test Acryl circle 2 mm cutter_v5 (Autodesk Fusion 360 design; units mm, degrees)
Autodesk Fusion 360 part; units mm, degrees
sketch "movingPlatform" plane through (0, 0, 0) normal (0, 0, 1) x (1, 0, 0)
  circle A0 centre (5.3745, -5.4565) radius 5
  line L0 (0, 0) -> (11, 0)
  line L1 (11, 0) -> (11, -11)
  line L2 (11, -11) -> (0, -11)
  line L3 (0, -11) -> (0, 0)
  dimension "d58" = 11
  dimension "d65" = 10
  dimension "d78" = 11
  constraint horizontal L0
  constraint vertical L1
  constraint horizontal L2
  constraint vertical L3
  measures "d58" distance of L0.start L2.end
  measures "d65" diameter of A0
  measures "d78" distance of L1 L3
extrude "Extrude15" add sketch "movingPlatform" along normal blind 3.2
